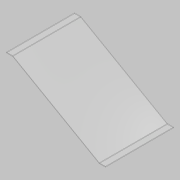
# Autodesk Inventor part: TemporaryLexan
Saved by Autodesk Inventor 2021 (Build 250183000, 183)
## iProperties
Created: 2021-03-03
Part Number: TemporaryLexan
Material: Generic
Document SubType Name: Modeling
Designer: Merkileg
Density: 1 g/cm^3
Appearance: Polycarbonate - Clear
Author: Merkileg
Autodesk Inventor part; units mm, degrees
ref_plane "YZ Plane" through (0, 0, 0) normal (1, 0, 0) x (0, 1, 0)
ref_plane "XZ Plane" through (0, 0, 0) normal (0, 1, 0) x (-1, 0, 0)
ref_plane "XY Plane" through (0, 0, 0) normal (0, 0, 1) x (1, 0, 0)
sketch "Sketch1" plane through (0, 0, 0) normal (0, 0, 1) x (1, 0, 0)
  line L0 (0, 0) -> (25.4, 0)
  line L1 (25.4, 0) -> (25.4, 2.9972)
  line L2 (25.4, 2.9972) -> (0, 2.9972)
  line L3 (-355.6, 206.1972) -> (0, 2.9972)
  line L4 (-355.6, 206.1972) -> (-381, 206.1972)
  line L5 (-381, 206.1972) -> (-381, 203.2)
  line L6 (-381, 203.2) -> (-355.6, 203.2)
  line L7 (-355.6, 203.2) -> (0, 0)
  dimension "d0" = 25.4
  dimension "d1" = 2.9972
  dimension "d2" = 25.4
  dimension "d3" = 25.4
  dimension "d4" = 2.9972
  dimension "d5" = 25.4
  constraints: 16 end point, 3 horizontal, 3 perpendicular, 1 parallel
  measures "d0" distance of L0.start L0.end
  measures "d1" distance of L0.end L1.end
  measures "d2" distance of L1.end L2.end
  measures "d3" distance of L3.start L4.end
  measures "d4" distance of L4.end L5.end
  measures "d5" distance of L5.end L6.end
extrude "Extrusion1" add sketch "Sketch1" along normal mid plane 279.4
body "Solid1"
